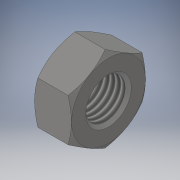
# Autodesk Inventor part: DIN 934 - M8x1(F)
Saved by Autodesk Inventor 2019 (Build 230136000, 136)
## iProperties
Created: 2023-04-07
Part Number: DIN 934 - M8x1(F)
Material: Generic
Catalog Web Link: www.cadenas.de
Description: DIN 934-Hex nut
Vendor: FESTO
Document SubType Name: Modeling
Designer: psAdmin
Manufacturer: FESTO
Mass: 0.695069 g
Surface Area: 6.2351 cm^2
Volume: 0.695069 cm^3
Density: 1 g/cm^3
Appearance: PSOLRGB-128-128-128
Category: PARTsolutions
Company: FESTO
Title: DIN 934 - M8x1(F)
Author: Cadenas PARTsolutions
Comments: Hex nut
PSOL_IDENT_0: {$CADENAS_DATA/23d-libs/festo/zyl_zubeh/din_934/din_934.prj},176 {VTYP=3D},{NB=DIN 934 - M8x1(F)},{L
PSOL_IDENT_1: INA=DIN 934 - M8x1(F)},{NN=DIN 934},{DATE=29.05.2015 05:51:25},{GEOMDATE=29.05.2015 05:51:14},{VERSI
PSOL_IDENT_2: ON=},{LINEID=120},{WBVAR=},{WBNUMERIC=}  {NB=DIN 934 - M8x1(F)},{LINA=DIN 934 - M8x1(F)},{KT=X},{IDN
PSOL_IDENT_3: R=},{NENN=M8x1},{D=8.000},{D1=6.773},{P=1.000},{M=6.500},{S=13.000}
NB: DIN 934 - M8x1(F)
NN: DIN 934
NT: Hex nut
NBSYN: DIN 934 - $NENN.(F)
LINA: DIN 934 - M8x1(F)
CATALOG: Festo
ROWDESC: M8x1
D: 8
D1: 6.773
P: 1
M: 6.5
S: 13
SUPPLIER: FESTO
ARTICLENO: DIN 934 - M8x1(F)
BOMINFO: DIN 934 - M8x1(F)
CREATOR: CADENAS GmbH
Autodesk Inventor part; units mm, degrees
sketch "Sketch_5" plane through (0, 0, 0) normal (0, 0, 1) x (1, 0, 0)
  line L0 (6.5, 0) -> (0, 0)
  line L1 (0, 0) -> (0, 6.4677)
  line L2 (0, 6.4677) -> (3.25, 12.0968)
  line L3 (3.25, 12.0968) -> (6.5, 6.4677)
  line L4 (6.5, 6.4677) -> (6.5, 0)
  line L5 (6.5, 0) -> (0, 0)
  constraints: 12 end point
revolve "Revolution1" add sketch "Sketch_5" angle 360 about axis through (6.5, 0, 0) along (1, 0, 0)
sketch "Sketch_2" plane through (0, 0, 0) normal (1, 0, 0) x (0, 1, 0)
  line L0 (26, 26) -> (-26, 26)
  line L1 (-26, 26) -> (-26, -26)
  line L2 (-26, -26) -> (26, -26)
  line L3 (26, -26) -> (26, 26)
  line L4 (-3.7528, 6.5) -> (-7.5056, 0)
  line L5 (-7.5056, 0) -> (-3.7528, -6.5)
  line L6 (-3.7528, -6.5) -> (3.7528, -6.5)
  line L7 (3.7528, -6.5) -> (7.5056, 0)
  line L8 (7.5056, 0) -> (3.7528, 6.5)
  line L9 (3.7528, 6.5) -> (-3.7528, 6.5)
  constraints: 20 end point
extrude "Extrusion1" cut sketch "Sketch_2" along normal mid plane 15
sketch "Sketch_4" plane through (0, 0, 0) normal (0, 0, 1) x (1, 0, 0)
  line L0 (6.5, 0) -> (0, 0)
  line L1 (0, 0) -> (0, 4)
  line L2 (0, 4) -> (0.5415, 3.4585)
  line L3 (0.5415, 3.4585) -> (5.9585, 3.4585)
  line L4 (5.9585, 3.4585) -> (6.5, 4)
  line L5 (6.5, 4) -> (6.5, 0)
  line L6 (6.5, 0) -> (0, 0)
  constraints: 14 end point
revolve "Revolution2" cut sketch "Sketch_4" angle 360 about axis through (6.5, 0, 0) along (1, 0, 0)
thread "Thread1" size "M8x1" class "6H" standard "ISO Metric profile" full length
ref_plane "IPoben_XY" through (6.5, 0, 0) normal (1, 0, 0) x (0, 0, -1)
ref_plane "IPoben_YZ" through (6.5, 0, 0) normal (0, 0, -1) x (0, 1, 0)
ref_plane "IPoben_ZX" through (6.5, 0, 0) normal (0, 1, 0) x (1, 0, 0)
ref_plane "IPunten_XY" through (0, 0, 0) normal (1, 0, 0) x (0, 0, -1)
ref_plane "IPunten_YZ" through (0, 0, 0) normal (0, 0, -1) x (0, 1, 0)
ref_plane "IPunten_ZX" through (0, 0, 0) normal (0, 1, 0) x (1, 0, 0)
body "Solid1"
